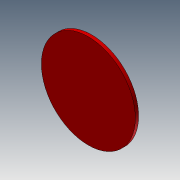
# Autodesk Inventor part: Manfrotto Logo 01 - 1
Saved by Autodesk Inventor 2011 (Build 150239000, 239)
## iProperties
Created: 2012-11-06
Part Number: Manfrotto Logo 01 - 1
Document SubType Name: Modeling
Designer: Lance
Density: 1 g/cm^3
Author: Lance
Autodesk Inventor part; units mm, degrees
ref_plane "YZ Plane" through (0, 0, 0) normal (1, 0, 0) x (0, 1, 0)
ref_plane "XZ Plane" through (0, 0, 0) normal (0, 1, 0) x (-1, 0, 0)
ref_plane "XY Plane" through (0, 0, 0) normal (0, 0, 1) x (1, 0, 0)
sketch "Sketch1" plane through (0, 0, 0) normal (0, 1, 0) x (-1, 0, 0)
  circle A0 centre (0, 0) radius 4.25
  dimension "d0" = 8.5
  constraints: 1 centre point, 1 coincident
  measures "d0" diameter of A0
extrude "Extrusion1" add sketch "Sketch1" along normal blind 0.3
sketch "Sketch2" plane through (0, 0.3, 0) normal (0, 1, 0) x (1, 0, 0)
  line L0 (-0.5, 0.5) -> (0.5, 0.5)
  line L1 (0.5, -1.5) -> (0.5, -4.25)
  line L2 (0.5, -4.25) -> (-0.5, -4.25)
  line L3 (-0.5, -4.25) -> (-0.5, -1.5)
  line L4 (-0.5, 0.5) -> (-2.7165, -3.3391)
  line L5 (-2.7165, -3.3391) -> (-1.8505, -3.8391)
  line L6 (-1.8505, -3.8391) -> (-0.5, -1.5)
  line L7 (0.5, -1.5) -> (1.8505, -3.8391)
  line L8 (1.8505, -3.8391) -> (2.7165, -3.3391)
  line L9 (2.7165, -3.3391) -> (0.5, 0.5)
  line L10 (0, 5.95) -> (0, -5.95) construction
  circle A0 centre (0, 0) radius 4.25 construction
  dimension "d3" = 60
  dimension "d4" = 1
  dimension "d5" = 0.5
  constraints: 20 end point, 4 perpendicular, 3 parallel, 3 tangent, 1 equal length, 1 horizontal, 1 point on line, 3 other
  measures "d3" angle of L9 L4
  measures "d4" distance between parallel lines of L1 L3
  measures "d5" distance from line of point (0, 0) L0
split_face "Split1"
sketch "Sketch3" plane through (-0.5, 0.3, -0.5) normal (0, 1, 0) x (1, 0, 0)
  line L0 (0, 1) -> (1, 1)
  line L1 (1, 1) -> (1, 3.75)
  line L2 (1, 3.75) -> (0, 3.75)
  line L3 (0, 3.75) -> (0, 1)
  line L4 (0, -4.7205) -> (0, -2) projected
  line L5 (1, -2) -> (1, -4.7205) projected
  arc A0 (3.1889, -3.7913) -> (-3.75, -0.5) centre (0.5, -0.5) ccw construction
  line L6 (0, 0) -> (1, 0) projected
  dimension "d6" = 1
  constraints: 8 end point, 2 collinear, 2 parallel, 1 horizontal, 1 perpendicular, 1 tangent
  measures "d6" distance between parallel lines of L6 L0
split_face "Split2"
body "Solid1"
